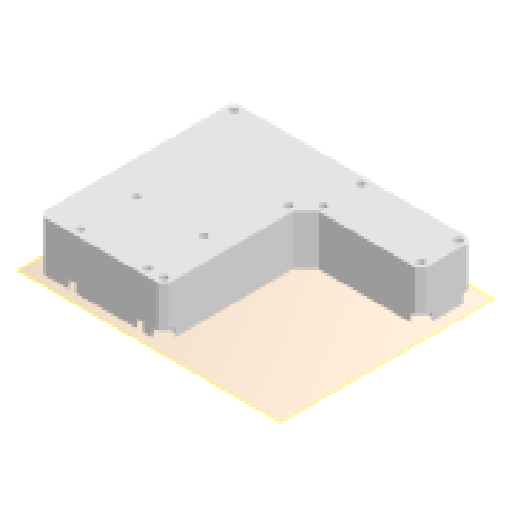
# Autodesk Inventor part: MIAB_Spacer
Saved by Autodesk Inventor 2024.1 (Build 281209000, 209)
## iProperties
Created: 2024-08-17
Part Number: MIAB_Spacer
Material: Generisch
Document SubType Name: Modeling
Designer: diederichbenedict
Density: 1 g/cm^3
Appearance: Vorgabe
Author: diederichbenedict
Autodesk Inventor part; units mm, degrees
ref_plane "YZ Plane" through (0, 0, 0) normal (1, 0, 0) x (0, 1, 0)
ref_plane "XZ Plane" through (0, 0, 0) normal (0, 1, 0) x (-1, 0, 0)
ref_plane "Arbeitsebene1" through (0, 0, 0) normal (0, 0, 1) x (1, 0, 0)
ref_plane "Arbeitsebene2" through (-65, -116.035, 20) normal (0, 0, -1) x (0, 1, 0)
sketch "Skizze1" plane through (0, 0, 0) normal (0, 0, 1) x (1, 0, 0)
  circle A0 centre (-21, -24.715) radius 10 projected
  circle A1 centre (-34.5, -13.465) radius 2 projected
  circle A2 centre (-7.5, -13.465) radius 2 projected
  circle A3 centre (-7.5, -35.965) radius 2 projected
  circle A4 centre (-34.5, -35.965) radius 2 projected
  circle A5 centre (-45, 35.965) radius 2 projected
  circle A6 centre (-1, -35.965) radius 2 projected
  circle A7 centre (-1, 14.0361) radius 2 projected
  circle A8 centre (45, 35.965) radius 2 projected
  circle A9 centre (45, 20.965) radius 2 projected
  circle A10 centre (5.9289, 20.965) radius 2 projected
  circle A11 centre (5.9289, 35.965) radius 2 projected
  line L0 (2, -38.965) -> (-48, -38.965) projected
  line L1 (-48, -38.965) -> (-48, 38.965) projected
  line L2 (-48, 38.965) -> (48, 38.965) projected
  line L3 (48, 38.965) -> (48, 17.965) projected
  line L4 (48, 17.965) -> (7.1716, 17.965) projected
  line L5 (7.1716, 17.965) -> (2, 12.7934) projected
  line L6 (2, 12.7934) -> (2, -38.965) projected
  point P0 (0, 0)
extrude "Extrusion1" add sketch "Skizze1" along normal up to surface (20 mm away) contours A0 | A1 | A2 | A3 | A4 | A5 | A6 | A7 | A8 | A9 | A10 | A11 | L0 L1 L2 L3 L4 L5 L6
chamfer "Fasen1" distance 2 angle 45 5 edges at (-48, 38.965, 10) (-48, -38.965, 10) (48, 38.965, 10) (48, 17.965, 10) (2, -38.965, 10)
sketch "Skizze2" plane through (0, 0, 0) normal (0, 0, -1) x (-1, 0, 0)
  circle A0 centre (21, -24.715) radius 10 projected
  circle A1 centre (34.5, -13.465) radius 2 projected
  circle A2 centre (7.5, -13.465) radius 2 projected
  circle A3 centre (7.5, -35.965) radius 2 projected
  circle A4 centre (34.5, -35.965) radius 2 projected
  circle A5 centre (45, 35.965) radius 2 projected
  circle A6 centre (1, -35.965) radius 2 projected
  circle A7 centre (1, 14.0361) radius 2 projected
  circle A8 centre (-45, 35.965) radius 2 projected
  circle A9 centre (-45, 20.965) radius 2 projected
  circle A10 centre (-5.9289, 20.965) radius 2 projected
  circle A11 centre (-5.9289, 35.965) radius 2 projected
  line L0 (-2, -38.965) -> (48, -38.965) projected
  line L1 (48, -38.965) -> (48, 38.965) projected
  line L2 (48, 38.965) -> (-48, 38.965) projected
  line L3 (-48, 38.965) -> (-48, 17.965) projected
  line L4 (-48, 17.965) -> (-7.1716, 17.965) projected
  line L5 (-7.1716, 17.965) -> (-2, 12.7934) projected
  line L6 (-2, 12.7934) -> (-2, -38.965) projected
  point P0 (0, 0)
hole "Bohrung1" at (45, 35.965, 0) at (5.9289, 35.965, 0) at (5.9289, 20.965, 0) at (-1, 14.0361, 0) at (45, 20.965, 0) at (-45, 35.965, 0) at (-7.5, -13.465, 0) at (-34.5, -13.465, 0) at (-34.5, -35.965, 0) at (-7.5, -35.965, 0) at (-1, -35.965, 0) direction (0, 0, 1) diameter 2.8 depth 20 counterbore diameter 6.5 counterbore depth 3.5
